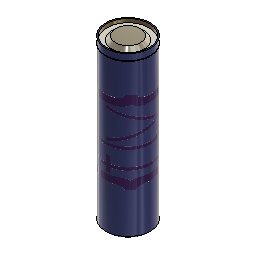
18650 (Autodesk Fusion 360 design; units mm, degrees)
Autodesk Fusion 360 part; units mm, degrees
sketch "Sketch1" plane through (0, 0, 0) normal (0, 1, 0) x (1, 0, 0)
  line L0 (4.9, 0) -> (4.9, -0.3)
  line L1 (4.9, -0.3) -> (5.1, -0.3)
  line L2 (5.1, -0.3) -> (5.1, 0)
  line L3 (0, 0) -> (4.9, 0)
  line L4 (5.1, 0) -> (8.3, 0)
  arc A0 (9, -0.7) -> (8.3, 0) centre (8.3, -0.7) ccw
  line L5 (9, -65) -> (8.5, -65)
  line L6 (8.5, -65) -> (8.5, -63.5)
  line L7 (8.5, -63.5) -> (6.5, -63.5)
  line L8 (6.5, -63.5) -> (5.0075, -64.9925)
  line L9 (5.0075, -64.9925) -> (0, -64.9925)
  line L10 (9, -62.5141) -> (8.5, -62.5141)
  line L11 (8.5, -62.5141) -> (8.5, -62.2467)
  line L12 (8.5, -62.2467) -> (9, -62.2467)
  line L13 (9, -0.7) -> (9, -62.2467)
  line L14 (9, -62.5141) -> (9, -65)
  line L15 (0, -64.9925) -> (0, 0)
  dimension "d11" = 9
  dimension "d12" = 0.7
  dimension "d13" = 0.3
  dimension "d14" = 135
  measures "d11" distance of L3.start
  measures "d12" radius of A0
  measures "d14" angle of L7 L8
revolve "Revolve1" add sketch "Sketch1" angle 360 about axis through (0, 0, 64.9925) along (0, 0, -1)
named bodies: "18650"
